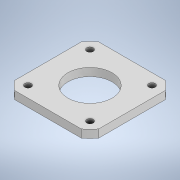
# Autodesk Inventor part: Spacer
Saved by Autodesk Inventor 2021 (Build 250183000, 183)
## iProperties
Created: 2022-09-01
Part Number: Spacer
Material: Ogólny
Document SubType Name: Modeling
Designer: MicnedSQ
Density: 1 g/cm^3
Appearance: Domyślna
Author: MicnedSQ
## iProperties of the stored document _Drukowanie 3D.ipt
Created: 2022-09-01
Part Number: _Drukowanie 3D
Material: Ogólny
Document SubType Name: Modeling
Designer: MicnedSQ
Density: 1 g/cm^3
Appearance: Domyślna
Author: MicnedSQ
Autodesk Inventor part; units mm, degrees
ref_plane "YZ Plane" through (0, 0, 0) normal (1, 0, 0) x (0, 1, 0)
ref_plane "XZ Plane" through (0, 0, 0) normal (0, 1, 0) x (-1, 0, 0)
ref_plane "XY Plane" through (0, 0, 0) normal (0, 0, 1) x (1, 0, 0)
sketch "Szkic1" plane through (0, 0, 0) normal (0, 1, 0) x (-1, 0, 0)
  line L0 (-16.7833, 21.15) -> (16.7833, 21.15)
  line L1 (21.15, 16.7833) -> (21.15, -16.7833)
  line L2 (16.7833, -21.15) -> (-16.7833, -21.15)
  line L3 (-21.15, -16.7833) -> (-21.15, 16.7833)
  line L4 (-21.15, 21.15) -> (21.15, -21.15) construction
  line L5 (21.15, 21.15) -> (-21.15, -21.15) construction
  circle A0 centre (15.6, 15.6) radius 1.65
  arc A1 (-16.7833, 21.15) -> (-21.15, 16.7833) centre (0, 0) ccw
  arc A2 (-21.15, -16.7833) -> (-16.7833, -21.15) centre (0, 0) ccw
  arc A3 (16.7833, -21.15) -> (21.15, -16.7833) centre (0, 0) ccw
  arc A4 (21.15, 16.7833) -> (16.7833, 21.15) centre (0, 0) ccw
  circle A5 centre (-15.6, 15.6) radius 1.65
  circle A6 centre (-15.6, -15.6) radius 1.65
  circle A7 centre (15.6, -15.6) radius 1.65
  circle A8 centre (0, 0) radius 11.1
  dimension "d0" = 42.3
  dimension "d1" = 42.3
  dimension "d2" = 15.6
  dimension "d3" = 3.3
  dimension "d7" = 360
  dimension "d11" = 22.2
  constraints: 12 end point, 9 centre point, 8 point on circle, 3 coincident, 2 midpoint, 2 parallel, 1 horizontal, 1 perpendicular, 1 point on line, 9 other
  measures "d0" distance of L4.end L5.end
  measures "d1" distance of L5.start L4.end
  measures "d2" horizontal distance of point (0, 0) point (15.6, 15.6)
  measures "d3" diameter of A0
  measures "d11" diameter of A8
extrude "Wyciągnięcie proste1" add sketch "Szkic1" along normal blind 4
